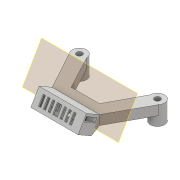
# Autodesk Inventor part: camera_holder_tarot_D435_30deg
Saved by Autodesk Inventor 2018 (Build 220112000, 112)
## iProperties
Created: 2018-09-04
Part Number: camera_holder_tarot_D435_30deg
Material: Generic
Document SubType Name: Modeling
Designer: Bardo91
Density: 1 g/cm^3
Appearance: Default
Author: Bardo91
Autodesk Inventor part; units mm, degrees
ref_plane "YZ Plane" through (0, 0, 0) normal (1, 0, 0) x (0, 1, 0)
ref_plane "XZ Plane" through (0, 0, 0) normal (0, 1, 0) x (-1, 0, 0)
ref_plane "XY Plane" through (0, 0, 0) normal (0, 0, 1) x (1, 0, 0)
sketch "Sketch1" plane through (0, 0, 0) normal (0, 0, 1) x (1, 0, 0)
  circle A0 centre (0, 0) radius 6
  line L0 (0, 0) -> (165, 0)
  circle A1 centre (165, 0) radius 6
  arc A2 (15, 0) -> (-11.6564, -9.4408) centre (0, 0) ccw
  arc A3 (176.6564, -9.4408) -> (150, 0) centre (165, 0) ccw
  line L1 (82.5, 0) -> (82.5, -90)
  line L2 (82.5, -90) -> (132.5, -90)
  line L3 (82.5, -90) -> (32.5, -90)
  line L4 (32.5, -90) -> (-11.6564, -9.4408)
  line L5 (132.5, -90) -> (176.6564, -9.4408)
  line L6 (82.5, -90) -> (82.5, -70)
  line L7 (82.5, -70) -> (112.5, -70)
  line L8 (82.5, -70) -> (52.5, -70)
  line L9 (112.5, -70) -> (150, 0)
  line L10 (52.5, -70) -> (15, 0)
  dimension "d0" = 12
  dimension "d1" = 165
  dimension "d2" = 12
  dimension "d3" = 30
  dimension "d4" = 30
  dimension "d5" = 90
  dimension "d6" = 50
  dimension "d7" = 50
  dimension "d8" = 20
  dimension "d9" = 30
  dimension "d10" = 30
  constraints: 22 end point, 4 centre point, 4 coincident, 4 horizontal, 4 point on circle, 2 point on line, 1 midpoint, 1 perpendicular, 1 vertical
  measures "d0" diameter of A0
  measures "d1" distance of L0.start L0.end
  measures "d2" diameter of A1
  measures "d3" diameter of A2
  measures "d4" diameter of A3
  measures "d5" distance of L1.start L1.end
  measures "d6" distance of L1.end L2.end
  measures "d7" distance of L1.end L3.end
  measures "d8" distance of L1.end L6.end
  measures "d9" distance of L6.end L7.end
  measures "d10" distance of L6.end L8.end
extrude "Extrusion1" add sketch "Sketch1" along normal blind 20 contours L10 L8 L1 L3 L4 A2 | A3 L5 L2 L1 L7 L9
sketch "Sketch2" plane through (0, 0, 20) normal (0, 0, 1) x (1, 0, 0)
  circle A0 centre (0, 0) radius 6
  circle A1 centre (0, 0) radius 15
  circle A2 centre (165, 0) radius 6 projected
  circle A3 centre (165, 0) radius 6
  circle A4 centre (165, 0) radius 15
  dimension "d13" = 12
  dimension "d14" = 30
  dimension "d15" = 12
  dimension "d16" = 30
  constraints: 4 centre point, 4 coincident
  measures "d13" diameter of A0
  measures "d14" diameter of A1
  measures "d15" diameter of A3
  measures "d16" diameter of A4
extrude "Extrusion2" add sketch "Sketch2" against normal blind 40
ref_plane "Work Plane1" through (32.5, -90, 20) normal (0, -0.8660254, 0.5) x (1, 0, 0)
sketch "Sketch3" plane through (32.5, -90, 20) normal (0, -0.8660254, 0.5) x (1, 0, 0)
  line L0 (0, 0) -> (100, 0) projected
  line L1 (100, 0) -> (100, -35)
  line L2 (100, -35) -> (0, -35)
  line L3 (0, -35) -> (0, 0)
  line L4 (100, -17.3205) -> (100, 0) projected
  line L5 (0, 0) -> (100, 0)
  point P0 (-32.5, 27.6795)
  dimension "d20" = 35
  dimension "d21" = 100
  constraints: 8 end point, 1 horizontal, 1 perpendicular, 1 vertical
  measures "d20" distance of L0.end L1.end
  measures "d21" distance of L1.end L2.end
extrude "Extrusion3" add sketch "Sketch3" along normal blind 32
sketch "Sketch4" plane through (132.5, -90, 20) normal (1, 0, 0) x (0, -0.5, -0.8660254)
  line L0 (0, 0) -> (-40.2796, 69.7663) projected
  line L1 (0, 0) -> (35, 0) projected
  line L2 (0, 0) -> (35, 0)
  line L3 (35, 0) -> (17.3205, 10)
  line L4 (17.3205, 10) -> (0, 0)
  point P0 (-27.6795, 87.9423)
  constraints: 6 end point, 1 horizontal
extrude "Extrusion4" add sketch "Sketch4" against normal up to surface (100 mm away)
sketch "Sketch5" plane through (132.5, -135.2128, 5.6891) normal (0, -0.5, -0.8660254) x (-1, 0, 0)
  line L0 (100, 32) -> (0, 32) projected
  line L1 (50, 32) -> (50, 0)
  line L2 (100, 0) -> (0, 0) projected
  line L3 (50, 16) -> (95, 16)
  line L4 (95, 16) -> (95, 29)
  line L5 (95, 29) -> (5, 29)
  line L6 (5, 29) -> (5, 3)
  line L7 (5, 3) -> (95, 3)
  line L8 (95, 3) -> (95, 16)
  point P0 (132.5, 119.9423)
  dimension "d26" = 45
  dimension "d27" = 13
  dimension "d28" = 90
  dimension "d29" = 26
  dimension "d30" = 90
  constraints: 14 end point, 4 perpendicular, 3 midpoint, 1 collinear, 1 horizontal, 1 point on line
  measures "d26" distance of L3.start L3.end
  measures "d27" distance of L3.end L4.end
  measures "d28" distance of L4.end L5.end
  measures "d29" distance of L5.end L6.end
  measures "d30" angle of L6 L5
extrude "Extrusion5" cut sketch "Sketch5" against normal blind 30
sketch "Sketch6" plane through (132.5, -90, 20) normal (1, 0, 0) x (0, 0, -1)
  line L0 (-10.1699, -27.6147) -> (2.8301, -5.0981) projected
  line L1 (-10.1699, -27.6147) -> (-2.3756, -32.1147)
  line L2 (-10.1699, -27.6147) -> (-1.1699, -27.6147) construction
  line L3 (-2.3756, -32.1147) -> (10.6244, -9.5981)
  line L4 (10.6244, -9.5981) -> (2.8301, -5.0981)
  line L5 (2.8301, -5.0981) -> (-10.1699, -27.6147)
  point P0 (20, 90)
  dimension "d33" = 9
  dimension "d34" = 30
  constraints: 10 end point, 4 perpendicular, 1 equal length, 1 horizontal
  measures "d33" distance of L0.start L1.end
  measures "d34" angle of L1 L2
extrude "Extrusion6" cut sketch "Sketch6" against normal through all
sketch "Sketch7" plane through (32.5, -117.7128, 36) normal (0, -0.8660254, 0.5) x (1, 0, 0)
  line L0 (5, -35) -> (95, -35) projected
  line L1 (50, -35) -> (50, 0)
  line L2 (100, 0) -> (0, 0) projected
  line L3 (50, -17.5) -> (47.5, -17.5)
  line L4 (47.5, -17.5) -> (47.5, -27.5)
  line L5 (47.5, -27.5) -> (52.5, -27.5)
  line L6 (52.5, -27.5) -> (52.5, -7.5)
  line L7 (52.5, -7.5) -> (47.5, -7.5)
  line L8 (47.5, -7.5) -> (47.5, -17.5)
  line L9 (50, -35) -> (60, -35)
  line L10 (60, -35) -> (70, -35)
  line L11 (70, -35) -> (95, -35)
  line L12 (60, -35) -> (60, -17.5)
  line L13 (60, -17.5) -> (57.5, -17.5)
  line L14 (57.5, -17.5) -> (57.5, -27.5)
  line L15 (57.5, -27.5) -> (62.5, -27.5)
  line L16 (62.5, -27.5) -> (62.5, -7.5)
  line L17 (62.5, -7.5) -> (57.5, -7.5)
  line L18 (57.5, -7.5) -> (57.5, -17.5)
  line L19 (70, -35) -> (70, -17.5)
  line L20 (70, -17.5) -> (67.5, -17.5)
  line L21 (67.5, -17.5) -> (67.5, -27.5)
  line L22 (67.5, -27.5) -> (72.5, -27.5)
  line L23 (72.5, -27.5) -> (72.5, -7.5)
  line L24 (72.5, -7.5) -> (67.5, -7.5)
  line L25 (67.5, -7.5) -> (67.5, -17.5)
  line L26 (70, -35) -> (80, -35)
  line L27 (80, -35) -> (80, -17.5)
  line L28 (80, -17.5) -> (77.5, -17.5)
  line L29 (77.5, -17.5) -> (77.5, -27.5)
  line L30 (77.5, -27.5) -> (82.5, -27.5)
  line L31 (82.5, -27.5) -> (82.5, -17.5)
  line L32 (82.5, -17.5) -> (82.5, -7.5)
  line L33 (82.5, -7.5) -> (77.5, -7.5)
  line L34 (77.5, -7.5) -> (77.5, -17.5)
  point P0 (-32.5, 27.6795)
  dimension "d37" = 2.5
  dimension "d38" = 10
  dimension "d39" = 5
  dimension "d40" = 20
  dimension "d41" = 10
  dimension "d42" = 10
  dimension "d44" = 2.5
  dimension "d45" = 10
  dimension "d46" = 5
  dimension "d47" = 20
  dimension "d48" = 2.5
  dimension "d49" = 10
  dimension "d50" = 5
  dimension "d51" = 10
  dimension "d52" = 2.5
  dimension "d53" = 10
  dimension "d54" = 5
  dimension "d55" = 10
  dimension "d56" = 10
  constraints: 66 end point, 20 perpendicular, 9 point on line, 3 midpoint, 2 collinear, 2 horizontal, 2 vertical
  measures "d37" distance of L3.start L3.end
  measures "d38" distance of L3.end L4.end
  measures "d39" distance of L4.end L5.end
  measures "d40" distance of L5.end L6.end
  measures "d41" distance of L1.start L9.end
  measures "d42" distance of L9.end L10.end
  measures "d44" distance of L12.end L13.end
  measures "d45" distance of L13.end L14.end
  measures "d46" distance of L14.end L15.end
  measures "d47" distance of L15.end L16.end
  measures "d48" distance of L19.end L20.end
  measures "d49" distance of L20.end L21.end
  measures "d50" distance of L21.end L22.end
  measures "d51" distance of L10.end L26.end
  measures "d52" distance of L27.end L28.end
  measures "d53" distance of L28.end L29.end
  measures "d54" distance of L29.end L30.end
  measures "d55" distance of L30.end L31.end
  measures "d56" distance of L31.end L32.end
extrude "Extrusion7" cut sketch "Sketch7" against normal through all
mirror "Mirror1" about plane through (80, -131.4628, 12.1843) normal (1, 0, 0) of "Extrusion7"
body "Solid1"
